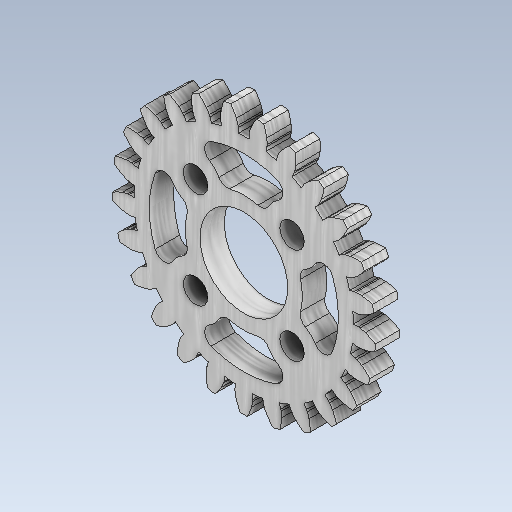
# Autodesk Inventor part: m2z25
Saved by Autodesk Inventor 2020 (Build 240168000, 168)
## iProperties
Created: 2020-02-27
Part Number: m2z25
Material: アルミニウム 7075
Document SubType Name: Modeling
Designer: tanjihayato
Density: 2.81 g/cm^3
Appearance: サテン - ブラシ仕上げ 重厚
Mass: 16.9382 g
Surface Area: 54.3595 cm^2
Volume: 6.02781 cm^3
Author: tanjihayato
Autodesk Inventor part; units mm, degrees
(part 1 of 2)
ref_plane "YZ Plane" through (0, 0, 0) normal (1, 0, 0) x (0, 1, 0)
ref_plane "XZ Plane" through (0, 0, 0) normal (0, 1, 0) x (-1, 0, 0)
ref_plane "XY Plane" through (0, 0, 0) normal (0, 0, 1) x (1, 0, 0)
sketch "スケッチ1" plane through (0, 0, 0) normal (0, 0, 1) x (1, 0, 0)
  arc A0 (24.5263, 48.3922) -> (24.4687, 48.0435) centre (26.7478, 47.8464) ccw
  arc A1 (24.8922, 49.4809) -> (24.5263, 48.3922) centre (30.6463, 46.941) ccw
  arc A2 (26.012, 51.446) -> (24.8922, 49.4809) centre (34.8467, 45.1102) ccw
  arc A3 (18.5668, 47.9382) -> (18.5978, 47.5862) centre (20.8543, 47.962) ccw
  arc A4 (18.6505, 49.0838) -> (18.5668, 47.9382) centre (24.8555, 48.0547) ccw
  arc A5 (19.2464, 51.2656) -> (18.6505, 49.0838) centre (29.3792, 47.3259) ccw
  arc A6 (12.9075, 46.0165) -> (13.025, 45.6833) centre (15.1172, 46.6084) ccw
  arc A7 (12.7036, 47.1469) -> (12.9075, 46.0165) centre (18.9696, 47.6932) ccw
  arc A8 (12.7382, 49.4083) -> (12.7036, 47.1469) centre (23.5324, 48.1123) ccw
  arc A9 (7.9038, 42.7477) -> (8.1005, 42.4542) centre (9.8969, 43.8706) ccw
  arc A10 (7.4253, 43.7919) -> (7.9038, 42.7477) centre (13.3585, 45.8793) ccw
  arc A11 (6.8964, 45.9909) -> (7.4253, 43.7919) centre (17.6738, 47.42) ccw
  arc A12 (3.8703, 38.3373) -> (4.1338, 38.1019) centre (5.5215, 39.9205) ccw
  arc A13 (3.1471, 39.2296) -> (3.8703, 38.3373) centre (8.3748, 42.727) ccw
  arc A14 (2.088, 41.228) -> (3.1471, 39.2296) centre (12.1714, 45.2925) ccw
  arc A15 (1.0604, 33.0623) -> (1.3741, 32.8998) centre (2.266, 35.0064) ccw
  arc A16 (0.138, 33.7468) -> (1.0604, 33.0623) centre (4.3317, 38.4344) ccw
  arc A17 (-1.3849, 35.4189) -> (0.138, 33.7468) centre (7.3709, 41.8634) ccw
  arc A18 (-0.3495, 27.2542) -> (-0.0052, 27.1749) centre (0.3348, 29.4371) ccw
  arc A19 (-1.4131, 27.6878) -> (-0.3495, 27.2542) centre (1.4831, 33.2711) ccw
  arc A20 (-3.304, 28.9287) -> (-1.4131, 27.6878) centre (3.5741, 37.3482) ccw
  arc A21 (-0.2706, 21.278) -> (0.0826, 21.2868) centre (-0.1508, 23.5625) ccw
  arc A22 (-1.4087, 21.4335) -> (-0.2706, 21.278) centre (0.008, 27.5616) ccw
  arc A23 (-3.5487, 22.1652) -> (-1.4087, 21.4335) centre (1.0194, 32.0306) ccw
  arc A24 (1.292, 15.5092) -> (1.6319, 15.6055) centre (0.8399, 17.7517) ccw
  arc A25 (0.151, 15.3767) -> (1.292, 15.5092) centre (-0.0008, 21.6646) ccw
  arc A26 (-2.1038, 15.5532) -> (0.151, 15.3767) centre (-0.1326, 26.2447) ccw
  arc A27 (4.2401, 10.3102) -> (4.5454, 10.488) centre (3.2446, 12.3698) ccw
  arc A28 (3.168, 9.8981) -> (4.2401, 10.3102) centre (1.4572, 15.9507) ccw
  arc A29 (0.9401, 9.5083) -> (3.168, 9.8981) centre (0.1905, 20.3542) ccw
  arc A30 (8.3886, 6.0077) -> (8.6401, 6.2559) centre (6.9121, 7.7551) ccw
  arc A31 (7.4526, 5.342) -> (8.3886, 6.0077) centre (4.2903, 10.7789) ccw
  arc A32 (5.3917, 4.4104) -> (7.4526, 5.342) centre (1.9683, 14.7291) ccw
  arc A33 (13.4767, 2.872) -> (13.6586, 3.175) centre (11.6121, 4.1973) ccw
  arc A34 (12.7357, 1.9945) -> (13.4767, 2.872) centre (8.3207, 6.4742) ccw
  arc A35 (10.9712, 0.5796) -> (12.7357, 1.9945) centre (5.0893, 9.7228) ccw
  arc A36 (19.1848, 1.1003) -> (19.2856, 1.439) centre (17.0492, 1.9202) ccw
  arc A37 (18.6853, 0.066) -> (19.1848, 1.1003) centre (13.2949, 3.307) ccw
  arc A38 (17.3281, -1.7432) -> (18.6853, 0.066) centre (9.3571, 5.6499) ccw
  arc A39 (25.1542, 0.8037) -> (25.1676, 1.1568) centre (22.8817, 1.0668) ccw
  arc A40 (24.9276, -0.3223) -> (25.1542, 0.8037) centre (18.9005, 1.4764) ccw
  arc A41 (24.0629, -2.4122) -> (24.9276, -0.3223) centre (14.5038, 2.7664) ccw
  arc A42 (31.0098, 2.001) -> (30.9349, 2.3464) centre (28.7433, 1.6907) ccw
  arc A43 (31.0703, 0.854) -> (31.0098, 2.001) centre (24.7853, 1.0973) ccw
  arc A44 (30.7526, -1.3853) -> (31.0703, 0.854) centre (20.2059, 1.2534) ccw
  arc A45 (36.3836, 4.6169) -> (36.2252, 4.9328) centre (34.2655, 3.7527) ccw
  arc A46 (36.7275, 3.521) -> (36.3836, 4.6169) centre (30.5794, 2.1936) ccw
  arc A47 (36.9766, 1.2731) -> (36.7275, 3.521) centre (26.1051, 1.2059) ccw
  arc A48 (40.9381, 8.487) -> (40.7062, 8.7536) centre (39.1015, 7.1232) ccw
  arc A49 (41.5437, 7.5111) -> (40.9381, 8.487) centre (35.9189, 4.6965) ccw
  arc A50 (42.3441, 5.3957) -> (41.5437, 7.5111) centre (31.8308, 2.6271) ccw
  arc A51 (44.387, 13.3682) -> (44.0961, 13.5688) centre (42.9473, 11.5905) ccw
  arc A52 (45.2163, 12.5736) -> (44.387, 13.3682) centre (40.4682, 8.4485) ccw
  arc A53 (46.5176, 10.7237) -> (45.2163, 12.5736) centre (37.0232, 5.4275) ccw
  arc A54 (46.5137, 18.9538) -> (46.182, 19.0757) centre (45.5613, 16.8739) ccw
  arc A55 (47.5146, 18.3903) -> (46.5137, 18.9538) centre (43.9415, 13.2141) ccw
  arc A56 (49.235, 16.9222) -> (47.5146, 18.3903) centre (41.356, 9.4312) ccw
  arc A57 (47.1845, 24.8928) -> (46.8329, 24.9283) centre (46.7792, 22.6413) ccw
  arc A58 (48.2941, 24.5959) -> (47.1845, 24.8928) centre (46.1205, 18.6937) ccw
  arc A59 (50.3256, 23.6018) -> (48.2941, 24.5959) centre (44.557, 14.3867) ccw
  arc A60 (46.3572, 30.812) -> (46.0079, 30.759) centre (46.5246, 28.5305) ccw
  arc A61 (47.5058, 30.8004) -> (46.3572, 30.812) centre (46.8683, 24.543) ccw
  arc A62 (49.7207, 30.3427) -> (47.5058, 30.8004) centre (46.425, 19.9825) ccw
  arc A63 (44.0839, 36.3395) -> (43.7587, 36.2013) centre (44.8135, 34.1713) ccw
  arc A64 (45.1993, 36.6139) -> (44.0839, 36.3395) centre (46.138, 30.3946) ccw
  arc A65 (47.4584, 36.7214) -> (45.1993, 36.6139) centre (46.8428, 25.8671) ccw
  arc A66 (40.5074, 41.128) -> (40.2268, 40.9132) centre (41.7532, 39.2093) ccw
  arc A67 (41.5195, 41.6712) -> (40.5074, 41.128) centre (43.9754, 35.8807) ccw
  arc A68 (43.6809, 42.3371) -> (41.5195, 41.6712) centre (45.784, 31.6707) ccw
  arc A69 (35.8524, 44.8766) -> (35.634, 44.5988) centre (37.5362, 43.3281) ccw
  arc A70 (36.6976, 45.6544) -> (35.8524, 44.8766) centre (40.5163, 40.6566) ccw
  arc A71 (38.6255, 46.837) -> (36.6976, 45.6544) centre (43.3151, 37.0287) ccw
  arc A72 (30.4114, 47.3498) -> (30.2689, 47.0264) centre (32.4274, 46.2687) ccw
  arc A73 (31.0366, 48.3133) -> (30.4114, 47.3498) centre (35.9783, 44.4223) ccw
  arc A74 (32.6099, 49.9382) -> (31.0366, 48.3133) centre (39.5914, 41.6043) ccw
  arc A75 (22.2177, 48.0435) -> (22.1602, 48.3922) centre (19.9386, 47.8464) ccw
  arc A76 (22.1602, 48.3922) -> (21.7942, 49.4809) centre (16.0401, 46.941) ccw
  arc A77 (21.7942, 49.4809) -> (20.6745, 51.446) centre (11.8398, 45.1102) ccw
  arc A78 (16.4175, 47.0264) -> (16.275, 47.3498) centre (14.259, 46.2687) ccw
  arc A79 (16.275, 47.3498) -> (15.6498, 48.3133) centre (10.7081, 44.4223) ccw
  arc A80 (15.6498, 48.3133) -> (14.0766, 49.9382) centre (7.0951, 41.6043) ccw
  arc A81 (11.0524, 44.5988) -> (10.834, 44.8766) centre (9.1502, 43.3281) ccw
  arc A82 (10.834, 44.8766) -> (9.9888, 45.6544) centre (6.1701, 40.6566) ccw
  arc A83 (9.9888, 45.6544) -> (8.0609, 46.837) centre (3.3713, 37.0287) ccw
  arc A84 (6.4596, 40.9132) -> (6.179, 41.128) centre (4.9332, 39.2093) ccw
  arc A85 (6.179, 41.128) -> (5.167, 41.6712) centre (2.7111, 35.8807) ccw
  arc A86 (5.167, 41.6712) -> (3.0055, 42.3371) centre (0.9025, 31.6707) ccw
  arc A87 (2.9277, 36.2013) -> (2.6025, 36.3395) centre (1.873, 34.1713) ccw
  arc A88 (2.6025, 36.3395) -> (1.4872, 36.6139) centre (0.5485, 30.3946) ccw
  arc A89 (1.4872, 36.6139) -> (-0.772, 36.7214) centre (-0.1564, 25.8671) ccw
  arc A90 (0.6786, 30.759) -> (0.3292, 30.812) centre (0.1618, 28.5305) ccw
  arc A91 (0.3292, 30.812) -> (-0.8194, 30.8004) centre (-0.1819, 24.543) ccw
  arc A92 (-0.8194, 30.8004) -> (-3.0343, 30.3427) centre (0.2614, 19.9825) ccw
  arc A93 (-0.1465, 24.9283) -> (-0.4981, 24.8928) centre (-0.0928, 22.6413) ccw
  arc A94 (-0.4981, 24.8928) -> (-1.6076, 24.5959) centre (0.5659, 18.6937) ccw
  arc A95 (-1.6076, 24.5959) -> (-3.6391, 23.6018) centre (2.1295, 14.3867) ccw
  arc A96 (0.5044, 19.0757) -> (0.1727, 18.9538) centre (1.1252, 16.8739) ccw
  arc A97 (0.1727, 18.9538) -> (-0.8282, 18.3903) centre (2.745, 13.2141) ccw
  arc A98 (-0.8282, 18.3903) -> (-2.5486, 16.9222) centre (5.3305, 9.4312) ccw
  arc A99 (2.5904, 13.5688) -> (2.2994, 13.3682) centre (3.7392, 11.5905) ccw
  arc A100 (2.2994, 13.3682) -> (1.4701, 12.5736) centre (6.2182, 8.4485) ccw
  arc A101 (1.4701, 12.5736) -> (0.1688, 10.7237) centre (9.6633, 5.4275) ccw
  arc A102 (5.9803, 8.7536) -> (5.7483, 8.487) centre (7.585, 7.1232) ccw
  arc A103 (5.7483, 8.487) -> (5.1427, 7.5111) centre (10.7675, 4.6965) ccw
  arc A104 (5.1427, 7.5111) -> (4.3423, 5.3957) centre (14.8556, 2.6271) ccw
  arc A105 (10.4612, 4.9328) -> (10.3028, 4.6169) centre (12.4209, 3.7527) ccw
  arc A106 (10.3028, 4.6169) -> (9.9589, 3.521) centre (16.107, 2.1936) ccw
  arc A107 (9.9589, 3.521) -> (9.7098, 1.2731) centre (20.5813, 1.2059) ccw
  arc A108 (15.7515, 2.3464) -> (15.6767, 2.001) centre (17.9432, 1.6907) ccw
  arc A109 (15.6767, 2.001) -> (15.6161, 0.854) centre (21.9012, 1.0973) ccw
  arc A110 (15.6161, 0.854) -> (15.9339, -1.3853) centre (26.4805, 1.2534) ccw
  arc A111 (21.5188, 1.1568) -> (21.5323, 0.8037) centre (23.8047, 1.0668) ccw
  arc A112 (21.5323, 0.8037) -> (21.7589, -0.3223) centre (27.7859, 1.4764) ccw
  arc A113 (21.7589, -0.3223) -> (22.6235, -2.4122) centre (32.1826, 2.7664) ccw
  arc A114 (27.4008, 1.439) -> (27.5016, 1.1003) centre (29.6373, 1.9202) ccw
  arc A115 (27.5016, 1.1003) -> (28.0011, 0.066) centre (33.3915, 3.307) ccw
  arc A116 (28.0011, 0.066) -> (29.3583, -1.7432) centre (37.3293, 5.6499) ccw
  arc A117 (33.0278, 3.175) -> (33.2097, 2.872) centre (35.0743, 4.1973) ccw
  arc A118 (33.2097, 2.872) -> (33.9507, 1.9945) centre (38.3658, 6.4742) ccw
  arc A119 (33.9507, 1.9945) -> (35.7152, 0.5796) centre (41.5972, 9.7228) ccw
  arc A120 (38.0463, 6.2559) -> (38.2978, 6.0077) centre (39.7743, 7.7551) ccw
  arc A121 (38.2978, 6.0077) -> (39.2338, 5.342) centre (42.3961, 10.7789) ccw
  arc A122 (39.2338, 5.342) -> (41.2948, 4.4104) centre (44.7181, 14.7291) ccw
  arc A123 (42.141, 10.488) -> (42.4463, 10.3102) centre (43.4418, 12.3698) ccw
  arc A124 (42.4463, 10.3102) -> (43.5185, 9.8981) centre (45.2292, 15.9507) ccw
  arc A125 (43.5185, 9.8981) -> (45.7463, 9.5083) centre (46.4959, 20.3542) ccw
  arc A126 (45.0545, 15.6055) -> (45.3945, 15.5092) centre (45.8465, 17.7517) ccw
  arc A127 (45.3945, 15.5092) -> (46.5354, 15.3767) centre (46.6872, 21.6646) ccw
  arc A128 (46.5354, 15.3767) -> (48.7902, 15.5532) centre (46.819, 26.2447) ccw
  arc A129 (46.6038, 21.2868) -> (46.9571, 21.278) centre (46.8372, 23.5625) ccw
  arc A130 (46.9571, 21.278) -> (48.0951, 21.4335) centre (46.6784, 27.5616) ccw
  arc A131 (48.0951, 21.4335) -> (50.2352, 22.1652) centre (45.667, 32.0306) ccw
  arc A132 (46.6916, 27.1749) -> (47.0359, 27.2542) centre (46.3517, 29.4371) ccw
  arc A133 (47.0359, 27.2542) -> (48.0995, 27.6878) centre (45.2034, 33.2711) ccw
  arc A134 (48.0995, 27.6878) -> (49.9904, 28.9287) centre (43.1124, 37.3482) ccw
  arc A135 (45.3123, 32.8998) -> (45.6261, 33.0623) centre (44.4205, 35.0064) ccw
  arc A136 (45.6261, 33.0623) -> (46.5484, 33.7468) centre (42.3548, 38.4344) ccw
  arc A137 (46.5484, 33.7468) -> (48.0713, 35.4189) centre (39.3155, 41.8634) ccw
  arc A138 (42.5526, 38.1019) -> (42.8161, 38.3373) centre (41.1649, 39.9205) ccw
  arc A139 (42.8161, 38.3373) -> (43.5393, 39.2296) centre (38.3116, 42.727) ccw
  arc A140 (43.5393, 39.2296) -> (44.5985, 41.228) centre (34.5151, 45.2925) ccw
  arc A141 (38.5859, 42.4542) -> (38.7826, 42.7477) centre (36.7895, 43.8706) ccw
  arc A142 (38.7826, 42.7477) -> (39.2611, 43.7919) centre (33.3279, 45.8793) ccw
  arc A143 (39.2611, 43.7919) -> (39.7901, 45.9909) centre (29.0127, 47.42) ccw
  arc A144 (33.6614, 45.6833) -> (33.779, 46.0165) centre (31.5692, 46.6084) ccw
  arc A145 (33.779, 46.0165) -> (33.9828, 47.1469) centre (27.7168, 47.6932) ccw
  arc A146 (33.9828, 47.1469) -> (33.9482, 49.4083) centre (23.154, 48.1123) ccw
  arc A147 (28.0887, 47.5862) -> (28.1196, 47.9382) centre (25.8321, 47.962) ccw
  arc A148 (28.1196, 47.9382) -> (28.0359, 49.0838) centre (21.831, 48.0547) ccw
  arc A149 (28.0359, 49.0838) -> (27.4401, 51.2656) centre (17.3073, 47.3259) ccw
  arc A150 (24.4212, 47.0524) -> (22.2653, 47.0524) centre (23.3432, 24.5782) ccw
  arc A151 (18.7982, 46.6144) -> (16.71, 46.0782) centre (23.3432, 24.5782) ccw
  arc A152 (13.4608, 44.7918) -> (11.5716, 43.7532) centre (23.3432, 24.5782) ccw
  arc A153 (8.7444, 41.6991) -> (7.1728, 40.2233) centre (23.3432, 24.5782) ccw
  arc A154 (4.9452, 37.5306) -> (3.7901, 35.7103) centre (23.3432, 24.5782) ccw
  arc A155 (2.3021, 32.5483) -> (1.6359, 30.4979) centre (23.3432, 24.5782) ccw
  arc A156 (0.9811, 27.0652) -> (0.8457, 24.9135) centre (23.3432, 24.5782) ccw
  arc A157 (1.0651, 21.4258) -> (1.4691, 19.3081) centre (23.3432, 24.5782) ccw
  arc A158 (2.549, 15.9845) -> (3.467, 14.0338) centre (23.3432, 24.5782) ccw
  arc A159 (5.3395, 11.0832) -> (6.7137, 9.4221) centre (23.3432, 24.5782) ccw
  arc A160 (9.2611, 7.0298) -> (11.0053, 5.7626) centre (23.3432, 24.5782) ccw
  arc A161 (14.0677, 4.0791) -> (16.0722, 3.2854) centre (23.3432, 24.5782) ccw
  arc A162 (19.457, 2.4164) -> (21.5959, 2.1462) centre (23.3432, 24.5782) ccw
  arc A163 (25.0905, 2.1462) -> (27.2294, 2.4164) centre (23.3432, 24.5782) ccw
  arc A164 (30.6142, 3.2854) -> (32.6188, 4.0791) centre (23.3432, 24.5782) ccw
  arc A165 (35.6811, 5.7626) -> (37.4253, 7.0298) centre (23.3432, 24.5782) ccw
  arc A166 (39.9727, 9.4221) -> (41.347, 11.0832) centre (23.3432, 24.5782) ccw
  arc A167 (43.2195, 14.0338) -> (44.1374, 15.9845) centre (23.3432, 24.5782) ccw
  arc A168 (45.2173, 19.3081) -> (45.6213, 21.4258) centre (23.3432, 24.5782) ccw
  arc A169 (45.8407, 24.9135) -> (45.7053, 27.0652) centre (23.3432, 24.5782) ccw
  arc A170 (45.0505, 30.4979) -> (44.3843, 32.5483) centre (23.3432, 24.5782) ccw
  arc A171 (42.8964, 35.7103) -> (41.7412, 37.5306) centre (23.3432, 24.5782) ccw
  arc A172 (39.5136, 40.2233) -> (37.942, 41.6991) centre (23.3432, 24.5782) ccw
  arc A173 (35.1148, 43.7532) -> (33.2256, 44.7918) centre (23.3432, 24.5782) ccw
  arc A174 (29.9764, 46.0782) -> (27.8882, 46.6144) centre (23.3432, 24.5782) ccw
  arc A175 (20.6745, 51.446) -> (19.2464, 51.2656) centre (23.3432, 24.5782) ccw
  arc A176 (14.0766, 49.9382) -> (12.7382, 49.4083) centre (23.3432, 24.5782) ccw
  arc A177 (8.0609, 46.837) -> (6.8964, 45.9909) centre (23.3432, 24.5782) ccw
  arc A178 (3.0055, 42.3371) -> (2.088, 41.228) centre (23.3432, 24.5782) ccw
  arc A179 (-0.772, 36.7214) -> (-1.3849, 35.4189) centre (23.3432, 24.5782) ccw
  arc A180 (-3.0343, 30.3427) -> (-3.304, 28.9287) centre (23.3432, 24.5782) ccw
  arc A181 (-3.6391, 23.6018) -> (-3.5487, 22.1652) centre (23.3432, 24.5782) ccw
  arc A182 (-2.5486, 16.9222) -> (-2.1038, 15.5532) centre (23.3432, 24.5782) ccw
  arc A183 (0.1688, 10.7237) -> (0.9401, 9.5083) centre (23.3432, 24.5782) ccw
  arc A184 (4.3423, 5.3957) -> (5.3917, 4.4104) centre (23.3432, 24.5782) ccw
  arc A185 (9.7098, 1.2731) -> (10.9712, 0.5796) centre (23.3432, 24.5782) ccw
  arc A186 (15.9339, -1.3853) -> (17.3281, -1.7432) centre (23.3432, 24.5782) ccw
  arc A187 (22.6235, -2.4122) -> (24.0629, -2.4122) centre (23.3432, 24.5782) ccw
  arc A188 (29.3583, -1.7432) -> (30.7526, -1.3853) centre (23.3432, 24.5782) ccw
  arc A189 (35.7152, 0.5796) -> (36.9766, 1.2731) centre (23.3432, 24.5782) ccw
  arc A190 (41.2948, 4.4104) -> (42.3441, 5.3957) centre (23.3432, 24.5782) ccw
  arc A191 (45.7463, 9.5083) -> (46.5176, 10.7237) centre (23.3432, 24.5782) ccw
  arc A192 (48.7902, 15.5532) -> (49.235, 16.9222) centre (23.3432, 24.5782) ccw
  arc A193 (50.2352, 22.1652) -> (50.3256, 23.6018) centre (23.3432, 24.5782) ccw
  arc A194 (49.9904, 28.9287) -> (49.7207, 30.3427) centre (23.3432, 24.5782) ccw
  arc A195 (48.0713, 35.4189) -> (47.4584, 36.7214) centre (23.3432, 24.5782) ccw
  arc A196 (44.5985, 41.228) -> (43.6809, 42.3371) centre (23.3432, 24.5782) ccw
  arc A197 (39.7901, 45.9909) -> (38.6255, 46.837) centre (23.3432, 24.5782) ccw
  arc A198 (33.9482, 49.4083) -> (32.6099, 49.9382) centre (23.3432, 24.5782) ccw
  arc A199 (27.4401, 51.2656) -> (26.012, 51.446) centre (23.3432, 24.5782) ccw
  line L0 (24.4212, 47.0524) -> (24.4687, 48.0435)
  line L1 (18.7982, 46.6144) -> (18.5978, 47.5862)
  line L2 (13.4608, 44.7918) -> (13.025, 45.6833)
  line L3 (8.7444, 41.6991) -> (8.1005, 42.4542)
  line L4 (4.9452, 37.5306) -> (4.1338, 38.1019)
  line L5 (2.3021, 32.5483) -> (1.3741, 32.8998)
  line L6 (0.9811, 27.0652) -> (-0.0052, 27.1749)
  line L7 (1.0651, 21.4258) -> (0.0826, 21.2868)
  line L8 (2.549, 15.9845) -> (1.6319, 15.6055)
  line L9 (5.3395, 11.0832) -> (4.5454, 10.488)
  line L10 (9.2611, 7.0298) -> (8.6401, 6.2559)
  line L11 (14.0677, 4.0791) -> (13.6586, 3.175)
  line L12 (19.457, 2.4164) -> (19.2856, 1.439)
  line L13 (25.0905, 2.1462) -> (25.1676, 1.1568)
  line L14 (30.6142, 3.2854) -> (30.9349, 2.3464)
  line L15 (35.6811, 5.7626) -> (36.2252, 4.9328)
  line L16 (39.9727, 9.4221) -> (40.7062, 8.7536)
  line L17 (43.2195, 14.0338) -> (44.0961, 13.5688)
  line L18 (45.2173, 19.3081) -> (46.182, 19.0757)
  line L19 (45.8407, 24.9135) -> (46.8329, 24.9283)
  line L20 (45.0505, 30.4979) -> (46.0079, 30.759)
  line L21 (42.8964, 35.7103) -> (43.7587, 36.2013)
  line L22 (39.5136, 40.2233) -> (40.2268, 40.9132)
  line L23 (35.1148, 43.7532) -> (35.634, 44.5988)
  line L24 (29.9764, 46.0782) -> (30.2689, 47.0264)
  line L25 (22.2653, 47.0524) -> (22.2177, 48.0435)
  line L26 (16.71, 46.0782) -> (16.4175, 47.0264)
  line L27 (11.5716, 43.7532) -> (11.0524, 44.5988)
  line L28 (7.1728, 40.2233) -> (6.4596, 40.9132)
  line L29 (3.7901, 35.7103) -> (2.9277, 36.2013)
  line L30 (1.6359, 30.4979) -> (0.6786, 30.759)
  line L31 (0.8457, 24.9135) -> (-0.1465, 24.9283)
  line L32 (1.4691, 19.3081) -> (0.5044, 19.0757)
  line L33 (3.467, 14.0338) -> (2.5904, 13.5688)
  line L34 (6.7137, 9.4221) -> (5.9803, 8.7536)
  line L35 (11.0053, 5.7626) -> (10.4612, 4.9328)
  line L36 (16.0722, 3.2854) -> (15.7515, 2.3464)
  line L37 (21.5959, 2.1462) -> (21.5188, 1.1568)
  line L38 (27.2294, 2.4164) -> (27.4008, 1.439)
  line L39 (32.6188, 4.0791) -> (33.0278, 3.175)
  line L40 (37.4253, 7.0298) -> (38.0463, 6.2559)
  line L41 (41.347, 11.0832) -> (42.141, 10.488)
  line L42 (44.1374, 15.9845) -> (45.0545, 15.6055)
  line L43 (45.6213, 21.4258) -> (46.6038, 21.2868)
  line L44 (45.7053, 27.0652) -> (46.6916, 27.1749)
  line L45 (44.3843, 32.5483) -> (45.3123, 32.8998)
  line L46 (41.7412, 37.5306) -> (42.5526, 38.1019)
  line L47 (37.942, 41.6991) -> (38.5859, 42.4542)
  line L48 (33.2256, 44.7918) -> (33.6614, 45.6833)
  line L49 (27.8882, 46.6144) -> (28.0887, 47.5862)
  line L50 (-5.6568, 24.5782) -> (52.3432, 24.5782)
  line L51 (23.3432, -4.4218) -> (23.3432, 53.5782)
  point P0 (0, 0)
  point P1 (0, 0)
  constraints: 300 point on circle, 150 centre point, 104 end point, 2 horizontal alignment, 148 other
extrude "押し出し1" add sketch "スケッチ1" along normal blind 5
sketch "スケッチ2" plane through (0, 0, 5) normal (0, 0, 1) x (1, 0, 0)
  arc A0 (22.1602, 48.3922) -> (21.7942, 49.4809) centre (16.0401, 46.941) ccw projected
  arc A1 (21.7942, 49.4809) -> (20.6745, 51.446) centre (11.8398, 45.1102) ccw projected
  arc A2 (20.6745, 51.446) -> (19.2464, 51.2656) centre (23.3432, 24.5782) ccw projected
  arc A3 (19.2464, 51.2656) -> (18.6505, 49.0838) centre (29.3792, 47.3259) ccw projected
  arc A4 (18.6505, 49.0838) -> (18.5668, 47.9382) centre (24.8555, 48.0547) ccw projected
  arc A5 (18.5668, 47.9382) -> (18.5978, 47.5862) centre (20.8543, 47.962) ccw projected
  line L0 (18.5978, 47.5862) -> (18.7982, 46.6144) projected
  arc A6 (18.7982, 46.6144) -> (16.71, 46.0782) centre (23.3432, 24.5782) ccw projected
  line L1 (16.71, 46.0782) -> (16.4175, 47.0264) projected
  arc A7 (16.4175, 47.0264) -> (16.275, 47.3498) centre (14.259, 46.2687) ccw projected
  arc A8 (16.275, 47.3498) -> (15.6498, 48.3133) centre (10.7081, 44.4223) ccw projected
  arc A9 (15.6498, 48.3133) -> (14.0766, 49.9382) centre (7.0951, 41.6043) ccw projected
  arc A10 (14.0766, 49.9382) -> (12.7382, 49.4083) centre (23.3432, 24.5782) ccw projected
  arc A11 (12.7382, 49.4083) -> (12.7036, 47.1469) centre (23.5324, 48.1123) ccw projected
  arc A12 (12.7036, 47.1469) -> (12.9075, 46.0165) centre (18.9696, 47.6932) ccw projected
  arc A13 (12.9075, 46.0165) -> (13.025, 45.6833) centre (15.1172, 46.6084) ccw projected
  line L2 (13.025, 45.6833) -> (13.4608, 44.7918) projected
  arc A14 (13.4608, 44.7918) -> (11.5716, 43.7532) centre (23.3432, 24.5782) ccw projected
  line L3 (11.5716, 43.7532) -> (11.0524, 44.5988) projected
  arc A15 (11.0524, 44.5988) -> (10.834, 44.8766) centre (9.1502, 43.3281) ccw projected
  arc A16 (10.834, 44.8766) -> (9.9888, 45.6544) centre (6.1701, 40.6566) ccw projected
  arc A17 (9.9888, 45.6544) -> (8.0609, 46.837) centre (3.3713, 37.0287) ccw projected
  arc A18 (8.0609, 46.837) -> (6.8964, 45.9909) centre (23.3432, 24.5782) ccw projected
  arc A19 (6.8964, 45.9909) -> (7.4253, 43.7919) centre (17.6738, 47.42) ccw projected
  arc A20 (7.4253, 43.7919) -> (7.9038, 42.7477) centre (13.3585, 45.8793) ccw projected
  arc A21 (7.9038, 42.7477) -> (8.1005, 42.4542) centre (9.8969, 43.8706) ccw projected
  line L4 (8.1005, 42.4542) -> (8.7444, 41.6991) projected
  arc A22 (8.7444, 41.6991) -> (7.1728, 40.2233) centre (23.3432, 24.5782) ccw projected
  line L5 (7.1728, 40.2233) -> (6.4596, 40.9132) projected
  arc A23 (6.4596, 40.9132) -> (6.179, 41.128) centre (4.9332, 39.2093) ccw projected
  arc A24 (6.179, 41.128) -> (5.167, 41.6712) centre (2.7111, 35.8807) ccw projected
  arc A25 (5.167, 41.6712) -> (3.0055, 42.3371) centre (0.9025, 31.6707) ccw projected
  arc A26 (3.0055, 42.3371) -> (2.088, 41.228) centre (23.3432, 24.5782) ccw projected
  arc A27 (2.088, 41.228) -> (3.1471, 39.2296) centre (12.1714, 45.2925) ccw projected
  arc A28 (3.1471, 39.2296) -> (3.8703, 38.3373) centre (8.3748, 42.727) ccw projected
  arc A29 (3.8703, 38.3373) -> (4.1338, 38.1019) centre (5.5215, 39.9205) ccw projected
  line L6 (4.1338, 38.1019) -> (4.9452, 37.5306) projected
  arc A30 (4.9452, 37.5306) -> (3.7901, 35.7103) centre (23.3432, 24.5782) ccw projected
  line L7 (3.7901, 35.7103) -> (2.9277, 36.2013) projected
  arc A31 (2.9277, 36.2013) -> (2.6025, 36.3395) centre (1.873, 34.1713) ccw projected
  arc A32 (2.6025, 36.3395) -> (1.4872, 36.6139) centre (0.5485, 30.3946) ccw projected
  arc A33 (1.4872, 36.6139) -> (-0.772, 36.7214) centre (-0.1564, 25.8671) ccw projected
  arc A34 (-0.772, 36.7214) -> (-1.3849, 35.4189) centre (23.3432, 24.5782) ccw projected
  arc A35 (-1.3849, 35.4189) -> (0.138, 33.7468) centre (7.3709, 41.8634) ccw projected
  arc A36 (0.138, 33.7468) -> (1.0604, 33.0623) centre (4.3317, 38.4344) ccw projected
  arc A37 (1.0604, 33.0623) -> (1.3741, 32.8998) centre (2.266, 35.0064) ccw projected
  line L8 (1.3741, 32.8998) -> (2.3021, 32.5483) projected
  arc A38 (2.3021, 32.5483) -> (1.6359, 30.4979) centre (23.3432, 24.5782) ccw projected
  line L9 (1.6359, 30.4979) -> (0.6786, 30.759) projected
  arc A39 (0.6786, 30.759) -> (0.3292, 30.812) centre (0.1618, 28.5305) ccw projected
  arc A40 (0.3292, 30.812) -> (-0.8194, 30.8004) centre (-0.1819, 24.543) ccw projected
  arc A41 (-0.8194, 30.8004) -> (-3.0343, 30.3427) centre (0.2614, 19.9825) ccw projected
  arc A42 (-3.0343, 30.3427) -> (-3.304, 28.9287) centre (23.3432, 24.5782) ccw projected
  arc A43 (-3.304, 28.9287) -> (-1.4131, 27.6878) centre (3.5741, 37.3482) ccw projected
  arc A44 (-1.4131, 27.6878) -> (-0.3495, 27.2542) centre (1.4831, 33.2711) ccw projected
  arc A45 (-0.3495, 27.2542) -> (-0.0052, 27.1749) centre (0.3348, 29.4371) ccw projected
  line L10 (-0.0052, 27.1749) -> (0.9811, 27.0652) projected
  arc A46 (0.9811, 27.0652) -> (0.8457, 24.9135) centre (23.3432, 24.5782) ccw projected
  line L11 (0.8457, 24.9135) -> (-0.1465, 24.9283) projected
  arc A47 (-0.1465, 24.9283) -> (-0.4981, 24.8928) centre (-0.0928, 22.6413) ccw projected
  arc A48 (-0.4981, 24.8928) -> (-1.6076, 24.5959) centre (0.5659, 18.6937) ccw projected
  arc A49 (-1.6076, 24.5959) -> (-3.6391, 23.6018) centre (2.1295, 14.3867) ccw projected
  arc A50 (-3.6391, 23.6018) -> (-3.5487, 22.1652) centre (23.3432, 24.5782) ccw projected
  arc A51 (-3.5487, 22.1652) -> (-1.4087, 21.4335) centre (1.0194, 32.0306) ccw projected
  arc A52 (-1.4087, 21.4335) -> (-0.2706, 21.278) centre (0.008, 27.5616) ccw projected
  arc A53 (-0.2706, 21.278) -> (0.0826, 21.2868) centre (-0.1508, 23.5625) ccw projected
  line L12 (0.0826, 21.2868) -> (1.0651, 21.4258) projected
  arc A54 (1.0651, 21.4258) -> (1.4691, 19.3081) centre (23.3432, 24.5782) ccw projected
  line L13 (1.4691, 19.3081) -> (0.5044, 19.0757) projected
  arc A55 (0.5044, 19.0757) -> (0.1727, 18.9538) centre (1.1252, 16.8739) ccw projected
  arc A56 (0.1727, 18.9538) -> (-0.8282, 18.3903) centre (2.745, 13.2141) ccw projected
  arc A57 (-0.8282, 18.3903) -> (-2.5486, 16.9222) centre (5.3305, 9.4312) ccw projected
  arc A58 (-2.5486, 16.9222) -> (-2.1038, 15.5532) centre (23.3432, 24.5782) ccw projected
  arc A59 (-2.1038, 15.5532) -> (0.151, 15.3767) centre (-0.1326, 26.2447) ccw projected
  arc A60 (0.151, 15.3767) -> (1.292, 15.5092) centre (-0.0008, 21.6646) ccw projected
  arc A61 (1.292, 15.5092) -> (1.6319, 15.6055) centre (0.8399, 17.7517) ccw projected
  line L14 (1.6319, 15.6055) -> (2.549, 15.9845) projected
  arc A62 (2.549, 15.9845) -> (3.467, 14.0338) centre (23.3432, 24.5782) ccw projected
  line L15 (3.467, 14.0338) -> (2.5904, 13.5688) projected
  arc A63 (2.5904, 13.5688) -> (2.2994, 13.3682) centre (3.7392, 11.5905) ccw projected
  arc A64 (2.2994, 13.3682) -> (1.4701, 12.5736) centre (6.2182, 8.4485) ccw projected
  arc A65 (1.4701, 12.5736) -> (0.1688, 10.7237) centre (9.6633, 5.4275) ccw projected
  arc A66 (0.1688, 10.7237) -> (0.9401, 9.5083) centre (23.3432, 24.5782) ccw projected
  arc A67 (0.9401, 9.5083) -> (3.168, 9.8981) centre (0.1905, 20.3542) ccw projected
  arc A68 (3.168, 9.8981) -> (4.2401, 10.3102) centre (1.4572, 15.9507) ccw projected
  arc A69 (4.2401, 10.3102) -> (4.5454, 10.488) centre (3.2446, 12.3698) ccw projected
  line L16 (4.5454, 10.488) -> (5.3395, 11.0832) projected
  arc A70 (5.3395, 11.0832) -> (6.7137, 9.4221) centre (23.3432, 24.5782) ccw projected
  line L17 (6.7137, 9.4221) -> (5.9803, 8.7536) projected
  arc A71 (5.9803, 8.7536) -> (5.7483, 8.487) centre (7.585, 7.1232) ccw projected
  arc A72 (5.7483, 8.487) -> (5.1427, 7.5111) centre (10.7675, 4.6965) ccw projected
  arc A73 (5.1427, 7.5111) -> (4.3423, 5.3957) centre (14.8556, 2.6271) ccw projected
  arc A74 (4.3423, 5.3957) -> (5.3917, 4.4104) centre (23.3432, 24.5782) ccw projected
  arc A75 (5.3917, 4.4104) -> (7.4526, 5.342) centre (1.9683, 14.7291) ccw projected
  arc A76 (7.4526, 5.342) -> (8.3886, 6.0077) centre (4.2903, 10.7789) ccw projected
  arc A77 (8.3886, 6.0077) -> (8.6401, 6.2559) centre (6.9121, 7.7551) ccw projected
  line L18 (8.6401, 6.2559) -> (9.2611, 7.0298) projected
  arc A78 (9.2611, 7.0298) -> (11.0053, 5.7626) centre (23.3432, 24.5782) ccw projected
  line L19 (11.0053, 5.7626) -> (10.4612, 4.9328) projected
  arc A79 (10.4612, 4.9328) -> (10.3028, 4.6169) centre (12.4209, 3.7527) ccw projected
  arc A80 (10.3028, 4.6169) -> (9.9589, 3.521) centre (16.107, 2.1936) ccw projected
  arc A81 (9.9589, 3.521) -> (9.7098, 1.2731) centre (20.5813, 1.2059) ccw projected
  arc A82 (9.7098, 1.2731) -> (10.9712, 0.5796) centre (23.3432, 24.5782) ccw projected
  arc A83 (10.9712, 0.5796) -> (12.7357, 1.9945) centre (5.0893, 9.7228) ccw projected
  arc A84 (12.7357, 1.9945) -> (13.4767, 2.872) centre (8.3207, 6.4742) ccw projected
  arc A85 (13.4767, 2.872) -> (13.6586, 3.175) centre (11.6121, 4.1973) ccw projected
  line L20 (13.6586, 3.175) -> (14.0677, 4.0791) projected
  arc A86 (14.0677, 4.0791) -> (16.0722, 3.2854) centre (23.3432, 24.5782) ccw projected
  line L21 (16.0722, 3.2854) -> (15.7515, 2.3464) projected
  arc A87 (15.7515, 2.3464) -> (15.6767, 2.001) centre (17.9432, 1.6907) ccw projected
  arc A88 (15.6767, 2.001) -> (15.6161, 0.854) centre (21.9012, 1.0973) ccw projected
  arc A89 (15.6161, 0.854) -> (15.9339, -1.3853) centre (26.4805, 1.2534) ccw projected
  arc A90 (15.9339, -1.3853) -> (17.3281, -1.7432) centre (23.3432, 24.5782) ccw projected
  arc A91 (17.3281, -1.7432) -> (18.6853, 0.066) centre (9.3571, 5.6499) ccw projected
  arc A92 (18.6853, 0.066) -> (19.1848, 1.1003) centre (13.2949, 3.307) ccw projected
  arc A93 (19.1848, 1.1003) -> (19.2856, 1.439) centre (17.0492, 1.9202) ccw projected
  line L22 (19.2856, 1.439) -> (19.457, 2.4164) projected
  arc A94 (19.457, 2.4164) -> (21.5959, 2.1462) centre (23.3432, 24.5782) ccw projected
  line L23 (21.5959, 2.1462) -> (21.5188, 1.1568) projected
  arc A95 (21.5188, 1.1568) -> (21.5323, 0.8037) centre (23.8047, 1.0668) ccw projected
  arc A96 (21.5323, 0.8037) -> (21.7589, -0.3223) centre (27.7859, 1.4764) ccw projected
  arc A97 (21.7589, -0.3223) -> (22.6235, -2.4122) centre (32.1826, 2.7664) ccw projected
  arc A98 (22.6235, -2.4122) -> (24.0629, -2.4122) centre (23.3432, 24.5782) ccw projected
  arc A99 (24.0629, -2.4122) -> (24.9276, -0.3223) centre (14.5038, 2.7664) ccw projected
  arc A100 (24.9276, -0.3223) -> (25.1542, 0.8037) centre (18.9005, 1.4764) ccw projected
  arc A101 (25.1542, 0.8037) -> (25.1676, 1.1568) centre (22.8817, 1.0668) ccw projected
  line L24 (25.1676, 1.1568) -> (25.0905, 2.1462) projected
  arc A102 (25.0905, 2.1462) -> (27.2294, 2.4164) centre (23.3432, 24.5782) ccw projected
  line L25 (27.2294, 2.4164) -> (27.4008, 1.439) projected
  arc A103 (27.4008, 1.439) -> (27.5016, 1.1003) centre (29.6373, 1.9202) ccw projected
  arc A104 (27.5016, 1.1003) -> (28.0011, 0.066) centre (33.3915, 3.307) ccw projected
  arc A105 (28.0011, 0.066) -> (29.3583, -1.7432) centre (37.3293, 5.6499) ccw projected
  arc A106 (29.3583, -1.7432) -> (30.7526, -1.3853) centre (23.3432, 24.5782) ccw projected
  arc A107 (30.7526, -1.3853) -> (31.0703, 0.854) centre (20.2059, 1.2534) ccw projected
  arc A108 (31.0703, 0.854) -> (31.0098, 2.001) centre (24.7853, 1.0973) ccw projected
  arc A109 (31.0098, 2.001) -> (30.9349, 2.3464) centre (28.7433, 1.6907) ccw projected
  line L26 (30.9349, 2.3464) -> (30.6142, 3.2854) projected
  arc A110 (30.6142, 3.2854) -> (32.6188, 4.0791) centre (23.3432, 24.5782) ccw projected
  line L27 (32.6188, 4.0791) -> (33.0278, 3.175) projected
  arc A111 (33.0278, 3.175) -> (33.2097, 2.872) centre (35.0743, 4.1973) ccw projected
  arc A112 (33.2097, 2.872) -> (33.9507, 1.9945) centre (38.3658, 6.4742) ccw projected
  arc A113 (33.9507, 1.9945) -> (35.7152, 0.5796) centre (41.5972, 9.7228) ccw projected
  arc A114 (35.7152, 0.5796) -> (36.9766, 1.2731) centre (23.3432, 24.5782) ccw projected
  arc A115 (36.9766, 1.2731) -> (36.7275, 3.521) centre (26.1051, 1.2059) ccw projected
  arc A116 (36.7275, 3.521) -> (36.3836, 4.6169) centre (30.5794, 2.1936) ccw projected
  arc A117 (36.3836, 4.6169) -> (36.2252, 4.9328) centre (34.2655, 3.7527) ccw projected
  line L28 (36.2252, 4.9328) -> (35.6811, 5.7626) projected
  arc A118 (35.6811, 5.7626) -> (37.4253, 7.0298) centre (23.3432, 24.5782) ccw projected
  line L29 (37.4253, 7.0298) -> (38.0463, 6.2559) projected
  arc A119 (38.0463, 6.2559) -> (38.2978, 6.0077) centre (39.7743, 7.7551) ccw projected
  arc A120 (38.2978, 6.0077) -> (39.2338, 5.342) centre (42.3961, 10.7789) ccw projected
  arc A121 (39.2338, 5.342) -> (41.2948, 4.4104) centre (44.7181, 14.7291) ccw projected
  arc A122 (41.2948, 4.4104) -> (42.3441, 5.3957) centre (23.3432, 24.5782) ccw projected
  arc A123 (42.3441, 5.3957) -> (41.5437, 7.5111) centre (31.8308, 2.6271) ccw projected
  arc A124 (41.5437, 7.5111) -> (40.9381, 8.487) centre (35.9189, 4.6965) ccw projected
  arc A125 (40.9381, 8.487) -> (40.7062, 8.7536) centre (39.1015, 7.1232) ccw projected
  line L30 (40.7062, 8.7536) -> (39.9727, 9.4221) projected
  arc A126 (39.9727, 9.4221) -> (41.347, 11.0832) centre (23.3432, 24.5782) ccw projected
  line L31 (41.347, 11.0832) -> (42.141, 10.488) projected
  arc A127 (42.141, 10.488) -> (42.4463, 10.3102) centre (43.4418, 12.3698) ccw projected
  arc A128 (42.4463, 10.3102) -> (43.5185, 9.8981) centre (45.2292, 15.9507) ccw projected
  arc A129 (43.5185, 9.8981) -> (45.7463, 9.5083) centre (46.4959, 20.3542) ccw projected
  arc A130 (45.7463, 9.5083) -> (46.5176, 10.7237) centre (23.3432, 24.5782) ccw projected
  arc A131 (46.5176, 10.7237) -> (45.2163, 12.5736) centre (37.0232, 5.4275) ccw projected
  arc A132 (45.2163, 12.5736) -> (44.387, 13.3682) centre (40.4682, 8.4485) ccw projected
  arc A133 (44.387, 13.3682) -> (44.0961, 13.5688) centre (42.9473, 11.5905) ccw projected
  line L32 (44.0961, 13.5688) -> (43.2195, 14.0338) projected
  arc A134 (43.2195, 14.0338) -> (44.1374, 15.9845) centre (23.3432, 24.5782) ccw projected
  line L33 (44.1374, 15.9845) -> (45.0545, 15.6055) projected
  arc A135 (45.0545, 15.6055) -> (45.3945, 15.5092) centre (45.8465, 17.7517) ccw projected
  arc A136 (45.3945, 15.5092) -> (46.5354, 15.3767) centre (46.6872, 21.6646) ccw projected
  arc A137 (46.5354, 15.3767) -> (48.7902, 15.5532) centre (46.819, 26.2447) ccw projected
  arc A138 (48.7902, 15.5532) -> (49.235, 16.9222) centre (23.3432, 24.5782) ccw projected
  arc A139 (49.235, 16.9222) -> (47.5146, 18.3903) centre (41.356, 9.4312) ccw projected
  arc A140 (47.5146, 18.3903) -> (46.5137, 18.9538) centre (43.9415, 13.2141) ccw projected
  arc A141 (46.5137, 18.9538) -> (46.182, 19.0757) centre (45.5613, 16.8739) ccw projected
  line L34 (46.182, 19.0757) -> (45.2173, 19.3081) projected
  arc A142 (45.2173, 19.3081) -> (45.6213, 21.4258) centre (23.3432, 24.5782) ccw projected
  line L35 (45.6213, 21.4258) -> (46.6038, 21.2868) projected
  arc A143 (46.6038, 21.2868) -> (46.9571, 21.278) centre (46.8372, 23.5625) ccw projected
  arc A144 (46.9571, 21.278) -> (48.0951, 21.4335) centre (46.6784, 27.5616) ccw projected
  arc A145 (48.0951, 21.4335) -> (50.2352, 22.1652) centre (45.667, 32.0306) ccw projected
  arc A146 (50.2352, 22.1652) -> (50.3256, 23.6018) centre (23.3432, 24.5782) ccw projected
  arc A147 (50.3256, 23.6018) -> (48.2941, 24.5959) centre (44.557, 14.3867) ccw projected
  arc A148 (48.2941, 24.5959) -> (47.1845, 24.8928) centre (46.1205, 18.6937) ccw projected
  arc A149 (47.1845, 24.8928) -> (46.8329, 24.9283) centre (46.7792, 22.6413) ccw projected
  line L36 (46.8329, 24.9283) -> (45.8407, 24.9135) projected
  arc A150 (45.8407, 24.9135) -> (45.7053, 27.0652) centre (23.3432, 24.5782) ccw projected
  line L37 (45.7053, 27.0652) -> (46.6916, 27.1749) projected
  arc A151 (46.6916, 27.1749) -> (47.0359, 27.2542) centre (46.3517, 29.4371) ccw projected
  arc A152 (47.0359, 27.2542) -> (48.0995, 27.6878) centre (45.2034, 33.2711) ccw projected
  arc A153 (48.0995, 27.6878) -> (49.9904, 28.9287) centre (43.1124, 37.3482) ccw projected
  arc A154 (49.9904, 28.9287) -> (49.7207, 30.3427) centre (23.3432, 24.5782) ccw projected
  arc A155 (49.7207, 30.3427) -> (47.5058, 30.8004) centre (46.425, 19.9825) ccw projected
  arc A156 (47.5058, 30.8004) -> (46.3572, 30.812) centre (46.8683, 24.543) ccw projected
  arc A157 (46.3572, 30.812) -> (46.0079, 30.759) centre (46.5246, 28.5305) ccw projected
  line L38 (46.0079, 30.759) -> (45.0505, 30.4979) projected
  arc A158 (45.0505, 30.4979) -> (44.3843, 32.5483) centre (23.3432, 24.5782) ccw projected
  line L39 (44.3843, 32.5483) -> (45.3123, 32.8998) projected
  arc A159 (45.3123, 32.8998) -> (45.6261, 33.0623) centre (44.4205, 35.0064) ccw projected
  arc A160 (45.6261, 33.0623) -> (46.5484, 33.7468) centre (42.3548, 38.4344) ccw projected
  arc A161 (46.5484, 33.7468) -> (48.0713, 35.4189) centre (39.3155, 41.8634) ccw projected
  arc A162 (48.0713, 35.4189) -> (47.4584, 36.7214) centre (23.3432, 24.5782) ccw projected
  arc A163 (47.4584, 36.7214) -> (45.1993, 36.6139) centre (46.8428, 25.8671) ccw projected
  arc A164 (45.1993, 36.6139) -> (44.0839, 36.3395) centre (46.138, 30.3946) ccw projected
  arc A165 (44.0839, 36.3395) -> (43.7587, 36.2013) centre (44.8135, 34.1713) ccw projected
  line L40 (43.7587, 36.2013) -> (42.8964, 35.7103) projected
  arc A166 (42.8964, 35.7103) -> (41.7412, 37.5306) centre (23.3432, 24.5782) ccw projected
  line L41 (41.7412, 37.5306) -> (42.5526, 38.1019) projected
  arc A167 (42.5526, 38.1019) -> (42.8161, 38.3373) centre (41.1649, 39.9205) ccw projected
  arc A168 (42.8161, 38.3373) -> (43.5393, 39.2296) centre (38.3116, 42.727) ccw projected
  arc A169 (43.5393, 39.2296) -> (44.5985, 41.228) centre (34.5151, 45.2925) ccw projected
  arc A170 (44.5985, 41.228) -> (43.6809, 42.3371) centre (23.3432, 24.5782) ccw projected
  arc A171 (43.6809, 42.3371) -> (41.5195, 41.6712) centre (45.784, 31.6707) ccw projected
  arc A172 (41.5195, 41.6712) -> (40.5074, 41.128) centre (43.9754, 35.8807) ccw projected
  arc A173 (40.5074, 41.128) -> (40.2268, 40.9132) centre (41.7532, 39.2093) ccw projected
  line L42 (40.2268, 40.9132) -> (39.5136, 40.2233) projected
  arc A174 (39.5136, 40.2233) -> (37.942, 41.6991) centre (23.3432, 24.5782) ccw projected
  line L43 (37.942, 41.6991) -> (38.5859, 42.4542) projected
  arc A175 (38.5859, 42.4542) -> (38.7826, 42.7477) centre (36.7895, 43.8706) ccw projected
  arc A176 (38.7826, 42.7477) -> (39.2611, 43.7919) centre (33.3279, 45.8793) ccw projected
  arc A177 (39.2611, 43.7919) -> (39.7901, 45.9909) centre (29.0127, 47.42) ccw projected
  arc A178 (39.7901, 45.9909) -> (38.6255, 46.837) centre (23.3432, 24.5782) ccw projected
  arc A179 (38.6255, 46.837) -> (36.6976, 45.6544) centre (43.3151, 37.0287) ccw projected
  arc A180 (36.6976, 45.6544) -> (35.8524, 44.8766) centre (40.5163, 40.6566) ccw projected
  arc A181 (35.8524, 44.8766) -> (35.634, 44.5988) centre (37.5362, 43.3281) ccw projected
  line L44 (35.634, 44.5988) -> (35.1148, 43.7532) projected
  arc A182 (35.1148, 43.7532) -> (33.2256, 44.7918) centre (23.3432, 24.5782) ccw projected
  line L45 (33.2256, 44.7918) -> (33.6614, 45.6833) projected
  arc A183 (33.6614, 45.6833) -> (33.779, 46.0165) centre (31.5692, 46.6084) ccw projected
  arc A184 (33.779, 46.0165) -> (33.9828, 47.1469) centre (27.7168, 47.6932) ccw projected
  arc A185 (33.9828, 47.1469) -> (33.9482, 49.4083) centre (23.154, 48.1123) ccw projected
  arc A186 (33.9482, 49.4083) -> (32.6099, 49.9382) centre (23.3432, 24.5782) ccw projected
  arc A187 (32.6099, 49.9382) -> (31.0366, 48.3133) centre (39.5914, 41.6043) ccw projected
  arc A188 (31.0366, 48.3133) -> (30.4114, 47.3498) centre (35.9783, 44.4223) ccw projected
  arc A189 (30.4114, 47.3498) -> (30.2689, 47.0264) centre (32.4274, 46.2687) ccw projected
  line L46 (30.2689, 47.0264) -> (29.9764, 46.0782) projected
  arc A190 (29.9764, 46.0782) -> (27.8882, 46.6144) centre (23.3432, 24.5782) ccw projected
  line L47 (27.8882, 46.6144) -> (28.0887, 47.5862) projected
  arc A191 (28.0887, 47.5862) -> (28.1196, 47.9382) centre (25.8321, 47.962) ccw projected
  arc A192 (28.1196, 47.9382) -> (28.0359, 49.0838) centre (21.831, 48.0547) ccw projected
  arc A193 (28.0359, 49.0838) -> (27.4401, 51.2656) centre (17.3073, 47.3259) ccw projected
  arc A194 (27.4401, 51.2656) -> (26.012, 51.446) centre (23.3432, 24.5782) ccw projected
  arc A195 (26.012, 51.446) -> (24.8922, 49.4809) centre (34.8467, 45.1102) ccw projected
  arc A196 (24.8922, 49.4809) -> (24.5263, 48.3922) centre (30.6463, 46.941) ccw projected
  arc A197 (24.5263, 48.3922) -> (24.4687, 48.0435) centre (26.7478, 47.8464) ccw projected
  line L48 (24.4687, 48.0435) -> (24.4212, 47.0524) projected
  arc A198 (24.4212, 47.0524) -> (22.2653, 47.0524) centre (23.3432, 24.5782) ccw projected
  line L49 (22.2653, 47.0524) -> (22.2177, 48.0435) projected
  arc A199 (22.2177, 48.0435) -> (22.1602, 48.3922) centre (19.9386, 47.8464) ccw projected
  circle A200 centre (23.3432, 24.5782) radius 9
  line L50 (13.4437, 34.4777) -> (33.2427, 34.4777) construction
  line L51 (33.2427, 34.4777) -> (33.2427, 14.6787) construction
  line L52 (33.2427, 14.6787) -> (13.4437, 14.6787) construction
  line L53 (13.4437, 14.6787) -> (13.4437, 34.4777) construction
  circle A201 centre (13.4437, 34.4777) radius 2.5
  circle A202 centre (33.2427, 34.4777) radius 2.5
  circle A203 centre (33.2427, 14.6787) radius 2.5
  circle A204 centre (13.4437, 14.6787) radius 2.5
  circle A205 centre (13.4437, 34.4777) radius 5 construction
  point P0 (0, 0)
  dimension "d2" = 18
  dimension "d3" = 5
  dimension "d4" = 5
  dimension "d5" = 5
  dimension "d6" = 5
  dimension "d7" = 10
  constraints: 8 end point, 7 coincident, 6 centre point, 1 horizontal, 1 tangent, 9 other
  measures "d2" diameter of A200
  measures "d3" diameter of A201
  measures "d4" diameter of A202
  measures "d5" diameter of A203
  measures "d6" diameter of A204
  measures "d7" diameter of A205
extrude "押し出し2" cut sketch "スケッチ2" against normal blind 5 contours A200 | A201 | A202 | A203 | A204